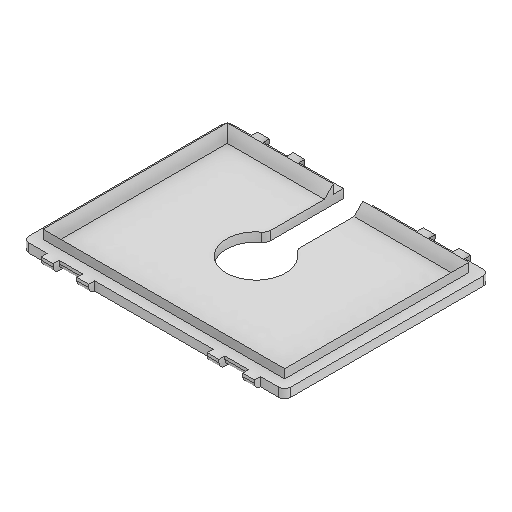
# Autodesk Inventor part: Janus wire holder lid
Saved by Autodesk Inventor 2025.1 (Build 291241020, 241B)
## iProperties
Created: 2025-03-14
Part Number: Janus wire holder lid
Material: Generic
Document SubType Name: Modeling
Designer: alexa
Density: 1 g/cm^3
Appearance: Default
Author: alexa
Autodesk Inventor part; units mm, degrees
ref_plane "YZ Plane" through (0, 0, 0) normal (1, 0, 0) x (0, 1, 0)
ref_plane "XZ Plane" through (0, 0, 0) normal (0, 1, 0) x (-1, 0, 0)
sketch "Sketch1" plane through (0, 0, 0) normal (0, 1, 0) x (-1, 0, 0)
  line L0 (0, 0) -> (-112.268, 0)
  line L1 (-112.268, 0) -> (-112.268, -87.63)
  line L2 (-112.268, -87.63) -> (0, -87.63)
  line L3 (0, -87.63) -> (0, 0)
  dimension "d0" = 87.63
  dimension "d1" = 112.268
  constraints: 8 end point, 2 parallel, 1 horizontal, 1 perpendicular
  measures "d0" distance of L0.end L1.end
  measures "d1" distance of L1.end L2.end
extrude "Extrusion1" add sketch "Sketch1" along normal blind 3.81
sketch "Sketch2" plane through (0, 3.81, 0) normal (0, 1, 0) x (1, 0, 0)
  line L0 (4.318, 83.312) -> (107.95, 83.312)
  line L1 (107.95, 83.312) -> (107.95, 4.318)
  line L2 (107.95, 4.318) -> (4.318, 4.318)
  line L3 (4.318, 4.318) -> (4.318, 83.312)
  line L4 (112.268, 87.63) -> (0, 87.63) projected
  line L5 (0, 87.63) -> (0, 0) projected
  line L6 (0, 0) -> (112.268, 0) projected
  line L7 (112.268, 0) -> (112.268, 87.63) projected
  line L8 (8.128, 79.502) -> (104.14, 79.502)
  line L9 (104.14, 79.502) -> (104.14, 8.128)
  line L10 (104.14, 8.128) -> (8.128, 8.128)
  line L11 (8.128, 8.128) -> (8.128, 79.502)
  dimension "d4" = 4.318
  dimension "d5" = 4.318
  dimension "d6" = 4.318
  dimension "d7" = 4.318
  dimension "d8" = 3.81
  constraints: 16 end point, 4 parallel, 2 perpendicular, 1 horizontal, 3 other
  measures "d4" distance between parallel lines of L4 L0
  measures "d5" distance between parallel lines of L5 L3
  measures "d6" distance between parallel lines of L6 L2
  measures "d7" distance between parallel lines of L7 L1
  measures "d8" distance between parallel lines of L3 L11
extrude "Extrusion2" add sketch "Sketch2" along normal blind 3.81 contours L0 L1 L2 L3
chamfer "Chamfer1" distance 3.81 angle 45 4 edges at (8.128, 7.62, -43.815) (56.134, 7.62, -79.502) (104.14, 7.62, -43.815) (56.134, 7.62, -8.128)
sketch "Sketch3" plane through (0, 0, 0) normal (0, -1, 0) x (1, 0, 0)
  arc A0 (63.754, -53.975) -> (48.514, -53.975) centre (56.134, -43.815) ccw
  line L0 (112.268, 0) -> (112.268, -87.63) projected
  line L1 (112.268, -87.63) -> (0, -87.63) projected
  line L2 (49.784, -56.515) -> (49.784, -87.63)
  line L3 (62.484, -56.515) -> (62.484, -87.63)
  arc A1 (49.784, -56.515) -> (48.514, -53.975) centre (46.609, -56.515) ccw
  arc A2 (63.754, -53.975) -> (62.484, -56.515) centre (65.659, -56.515) ccw
  point P0 (0, 0)
  point P1 (112.268, -43.815)
  point P2 (56.134, -87.63)
  point P3 (43.434, -43.815)
  point P4 (43.434, -87.63)
  point P5 (68.834, -43.815)
  point P6 (68.834, -87.63)
  point P7 (49.784, -54.8135)
  point P8 (62.484, -54.8135)
  point P9 (56.134, -87.63)
  dimension "d14" = 25.4
  dimension "d17" = 12.7
  dimension "d18" = 6.35
  dimension "d19" = 3.175
  constraints: 10 point on circle, 6 point on line, 4 end point, 4 tangent, 3 centre point, 3 midpoint, 2 perpendicular, 1 equal radius, 1 horizontal alignment, 1 vertical alignment
  measures "d14" diameter of A0
  measures "d17" distance between parallel lines of L3 L2
  measures "d18" distance from line of point (56.134, -87.63) L3
  measures "d19" radius of A1
extrude "Extrusion3" cut sketch "Sketch3" against normal blind 62.865
fillet "Fillet1" radius 2.54 4 edges at (0, 1.905, -87.63) (112.268, 1.905, -87.63) (112.268, 1.905, 0) (0, 1.905, 0)
sketch "Sketch4" plane through (49.784, 0, -87.63) normal (0, 0, -1) x (-1, 0, 0)
  line L0 (0, 0) -> (47.244, 0) projected
  line L1 (45.466, 3.81) -> (0, 3.81) projected
  line L2 (39.37, 0) -> (34.29, 0)
  line L3 (34.29, 0) -> (34.29, 3.81)
  line L4 (34.29, 3.81) -> (39.37, 3.81)
  line L5 (39.37, 3.81) -> (39.37, 0)
  line L6 (24.13, 3.81) -> (19.05, 3.81)
  line L7 (19.05, 3.81) -> (19.05, 0)
  line L8 (19.05, 0) -> (24.13, 0)
  line L9 (24.13, 0) -> (24.13, 3.81)
  line L10 (-31.75, 3.81) -> (-36.83, 3.81)
  line L11 (-36.83, 3.81) -> (-36.83, 0)
  line L12 (-36.83, 0) -> (-31.75, 0)
  line L13 (-31.75, 0) -> (-31.75, 3.81)
  line L14 (-12.7, 3.81) -> (-58.166, 3.81) projected
  line L15 (-46.99, 3.81) -> (-52.07, 3.81)
  line L16 (-52.07, 3.81) -> (-52.07, 0)
  line L17 (-52.07, 0) -> (-46.99, 0)
  line L18 (-46.99, 0) -> (-46.99, 3.81)
  line L19 (45.466, 7.62) -> (-58.166, 7.62) projected
  point P0 (49.784, 0)
  point P1 (34.29, 1.905)
  point P2 (39.37, 1.905)
  point P3 (19.05, 1.905)
  point P4 (24.13, 1.905)
  point P5 (-36.83, 1.905)
  point P6 (-31.75, 1.905)
  point P7 (-52.07, 1.905)
  point P8 (-46.99, 1.905)
  point P9 (-6.35, 7.62)
  point P10 (-52.07, 3.81)
  point P11 (19.05, 3.81)
  point P12 (19.05, 0)
  dimension "d21" = 5.08
  dimension "d22" = 5.08
  dimension "d23" = 5.08
  dimension "d24" = 5.08
  dimension "d25" = 10.16
  dimension "d26" = 10.16
  dimension "d27" = 50.8
  dimension "d28" = 25.4
  constraints: 32 end point, 9 midpoint, 8 parallel, 8 point on line, 4 horizontal, 4 perpendicular
  measures "d21" distance of point (34.29, 1.905) point (39.37, 1.905)
  measures "d22" distance of point (19.05, 1.905) point (24.13, 1.905)
  measures "d23" distance of point (-36.83, 1.905) point (-31.75, 1.905)
  measures "d24" distance of point (-52.07, 1.905) point (-46.99, 1.905)
  measures "d25" distance of point (-46.99, 1.905) point (-36.83, 1.905)
  measures "d26" distance of point (34.29, 1.905) point (24.13, 1.905)
  measures "d27" distance of point (-31.75, 1.905) point (19.05, 1.905)
  measures "d28" horizontal distance of point (-6.35, 7.62) point (19.05, 1.905)
extrude "Extrusion4" add sketch "Sketch4" along normal blind 2.54 contours L7 L1 L9 L0 | L3 L1 L5 L0 | L13 L12 L11 L10 | L18 L17 L16 L14
ref_plane "Work Plane1" through (49.784, 0, -43.815) normal (0, 0, -1) x (-1, 0, 0)
mirror "Mirror1" about plane through (49.784, 0, -43.815) normal (0, 0, -1) of "Extrusion4"
fillet "Fillet2" radius 2.54 12 edges at (12.954, 0, -90.17) (20.574, 0, -87.63) (28.194, 0, -90.17) (91.694, 0, -87.63) (99.314, 0, -90.17) (84.074, 0, 2.54) (91.694, 0, 0) (99.314, 0, 2.54) (12.954, 0, 2.54) (20.574, 0, 0) (28.194, 0, 2.54) (84.074, 0, -90.17)
equation "\"d5\" = d4"
equation "\"d6\" = d4"
equation "\"d7\" = d4"
equation "\"d18\" = 0.5 * d17"
equation "\"d22\" = d21"
equation "\"d23\" = d22"
equation "\"d24\" = d23"
equation "\"d26\" = d25"
equation "\"d28\" = 0.5 * d27"
body "Solid1"
